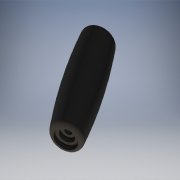
# Autodesk Inventor part: roller
Saved by Autodesk Inventor 2018 (Build 220112000, 112)
## iProperties
Created: 2023-12-05
Part Number: roller
Material: Rubber
Document SubType Name: Modeling
Designer: DDUGKY
Density: 0.93 g/cm^3
Appearance: Rubber - Black
Author: DDUGKY
Autodesk Inventor part; units mm, degrees
ref_plane "YZ Plane" through (0, 0, 0) normal (1, 0, 0) x (0, 1, 0)
ref_plane "XZ Plane" through (0, 0, 0) normal (0, 1, 0) x (-1, 0, 0)
ref_plane "XY Plane" through (0, 0, 0) normal (0, 0, 1) x (1, 0, 0)
sketch "Sketch1" plane through (0, 0, 0) normal (1, 0, 0) x (0, 1, 0)
  line L0 (0, 25.5) -> (0, -25.5)
  line L1 (0, 25.5) -> (8.33, 25.5)
  line L2 (0, -25.5) -> (8.33, -25.5)
  arc A0 (8.33, -25.5) -> (8.33, 25.5) centre (-164.8022, 0) ccw
  point P0 (0, 0)
  dimension "d0" = 51
  dimension "d1" = 8.33
  dimension "d2" = 8.33
  dimension "d3" = 175
  constraints: 6 end point, 2 horizontal, 2 point on circle, 1 centre point, 1 vertical
  measures "d0" distance of L0.start L0.end
  measures "d1" distance of L0.start L1.end
  measures "d2" distance of L0.end L2.end
  measures "d3" radius of A0
revolve "Revolution1" add sketch "Sketch1" angle 360 about axis through (0, 0, 25.5) along (0, 0, -1)
sketch "Sketch2" plane through (0, 0, 25.5) normal (0, 0, 1) x (1, 0, 0)
  circle A0 centre (0, 0) radius 6
  dimension "d5" = 12
  constraints: 1 centre point, 1 coincident
  measures "d5" diameter of A0
extrude "Extrusion1" cut sketch "Sketch2" against normal blind 2
sketch "Sketch3" plane through (0, 0, 23.5) normal (0, 0, 1) x (1, 0, 0)
  circle A0 centre (0, 0) radius 4
  dimension "d8" = 8
  constraints: 1 centre point, 1 coincident
  measures "d8" diameter of A0
extrude "Extrusion2" cut sketch "Sketch3" against normal blind 2
fillet "Fillet1" radius 2.5 1 edges at (0, -8.33, 25.5)
mirror "Mirror1" about plane through (0, 0, 0) normal (0, 0, 1) of "Extrusion1", "Extrusion2", "Fillet1"
sketch "Sketch4" plane through (0, 0, 0) normal (0, 0, 1) x (1, 0, 0)
  circle A0 centre (0, 0) radius 4 projected
  circle A1 centre (0, 0) radius 2
  point P0 (0, 0)
  dimension "d12" = 4
  constraints: 1 centre point, 1 coincident
  measures "d12" diameter of A1
extrude "Extrusion3" cut sketch "Sketch4" along normal mid plane 805.5 contours A1
sketch "Sketch5" plane through (0, 0, 0) normal (1, 0, 0) x (0, 1, 0)
  line L0 (-0.25, -20) -> (0.25, -20)
  line L1 (0.25, -20) -> (0.25, 20)
  line L2 (0.25, 20) -> (-0.25, 20)
  line L3 (-0.25, 20) -> (-0.25, -20)
  line L4 (-0.25, -20) -> (0.25, 20) construction
  line L5 (0.25, -20) -> (-0.25, 20) construction
  point P0 (0, 0)
  dimension "d17" = 0.5
  dimension "d18" = 40
  constraints: 12 end point, 2 midpoint, 2 parallel, 1 horizontal, 1 perpendicular
  measures "d17" distance of L1.end L2.end
  measures "d18" distance of L0.end L1.end
extrude "Extrusion4" cut sketch "Sketch5" along normal mid plane 40
body "Solid1"
